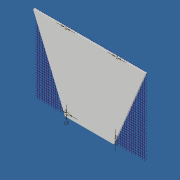
# Autodesk Inventor part: Detektorplatine
Saved by Autodesk Inventor 2018 (Build 220112000, 112)
## iProperties
Created: 2018-11-01
Part Number: Detektorplatine
Material: Generisch
Document SubType Name: Modeling
Designer: M.Knabel
Density: 1 g/cm^3
Appearance: Vorgabe
Author: M.Knabel
Autodesk Inventor part; units mm, degrees
ref_plane "YZ Plane" through (0, 0, 0) normal (1, 0, 0) x (0, 1, 0)
ref_plane "XZ Plane" through (0, 0, 0) normal (0, 1, 0) x (-1, 0, 0)
ref_plane "XY Plane" through (0, 0, 0) normal (0, 0, 1) x (1, 0, 0)
sketch "Skizze1" plane through (0, 0, 0) normal (0, 1, 0) x (-1, 0, 0)
  line L0 (-50.2277, 69) -> (50.2277, 69)
  line L1 (50.2277, 69) -> (21.647, 0)
  line L2 (21.647, 0) -> (-21.647, 0)
  line L3 (-21.647, 0) -> (-50.2277, 69)
  line L4 (0, -13.8) -> (0, 82.8) construction
  line L5 (70.3188, 0) -> (-70.3188, 0) construction
  point P0 (0, 0)
  dimension "d0" = 43.294
  dimension "d1" = 112.5
  dimension "d2" = 69
  constraints: 8 end point, 1 collinear, 1 horizontal, 1 parallel, 1 other
  measures "d0" distance of L1.end L2.end
  measures "d1" angle of L2 L3
  measures "d2" distance between parallel lines of L2 L0
extrude "Extrusion1" add sketch "Skizze1" along normal blind 1.5
sketch "Skizze2" plane through (0, 1.5, 0) normal (0, 1, 0) x (1, 0, 0)
  line L0 (21.647, 0) -> (-21.647, 0) projected
  line L1 (-21.647, 0) -> (-21.647, 7.3765) construction
  point P0 (0, 0)
  point P1 (-21.647, -1.5)
  point P2 (-19.647, -1.5)
  point P3 (-17.647, -1.5)
  point P4 (-15.647, -1.5)
  point P5 (-13.647, -1.5)
  point P6 (-11.647, -1.5)
  point P7 (-9.647, -1.5)
  point P8 (-7.647, -1.5)
  point P9 (-5.647, -1.5)
  point P10 (-3.647, -1.5)
  point P11 (-1.647, -1.5)
  point P12 (0.353, -1.5)
  point P13 (2.353, -1.5)
  point P14 (4.353, -1.5)
  point P15 (6.353, -1.5)
  point P16 (8.353, -1.5)
  point P17 (10.353, -1.5)
  point P18 (12.353, -1.5)
  point P19 (14.353, -1.5)
  point P20 (16.353, -1.5)
  point P21 (18.353, -1.5)
  point P22 (20.353, -1.5)
  point P23 (22.353, -1.5)
  point P24 (22.353, -3.5)
  point P25 (20.353, -3.5)
  point P26 (18.353, -3.5)
  point P27 (16.353, -3.5)
  point P28 (14.353, -3.5)
  point P29 (12.353, -3.5)
  point P30 (10.353, -3.5)
  point P31 (8.353, -3.5)
  point P32 (6.353, -3.5)
  point P33 (4.353, -3.5)
  point P34 (2.353, -3.5)
  point P35 (0.353, -3.5)
  point P36 (-1.647, -3.5)
  point P37 (-3.647, -3.5)
  point P38 (-5.647, -3.5)
  point P39 (-7.647, -3.5)
  point P40 (-9.647, -3.5)
  point P41 (-11.647, -3.5)
  point P42 (-13.647, -3.5)
  point P43 (-15.647, -3.5)
  point P44 (-17.647, -3.5)
  point P45 (-19.647, -3.5)
  point P46 (-21.647, -3.5)
  point P47 (22.353, -5.5)
  point P48 (20.353, -5.5)
  point P49 (18.353, -5.5)
  point P50 (16.353, -5.5)
  point P51 (14.353, -5.5)
  point P52 (12.353, -5.5)
  point P53 (10.353, -5.5)
  point P54 (8.353, -5.5)
  point P55 (6.353, -5.5)
  point P56 (4.353, -5.5)
  point P57 (2.353, -5.5)
  point P58 (0.353, -5.5)
  point P59 (-1.647, -5.5)
  point P60 (-3.647, -5.5)
  point P61 (-5.647, -5.5)
  point P62 (-7.647, -5.5)
  point P63 (-9.647, -5.5)
  point P64 (-11.647, -5.5)
  point P65 (-13.647, -5.5)
  point P66 (-15.647, -5.5)
  point P67 (-17.647, -5.5)
  point P68 (-19.647, -5.5)
  point P69 (-21.647, -5.5)
  point P70 (22.353, -7.5)
  point P71 (20.353, -7.5)
  point P72 (18.353, -7.5)
  point P73 (16.353, -7.5)
  point P74 (14.353, -7.5)
  point P75 (12.353, -7.5)
  point P76 (10.353, -7.5)
  point P77 (8.353, -7.5)
  point P78 (6.353, -7.5)
  point P79 (4.353, -7.5)
  point P80 (2.353, -7.5)
  point P81 (0.353, -7.5)
  point P82 (-1.647, -7.5)
  point P83 (-3.647, -7.5)
  point P84 (-5.647, -7.5)
  point P85 (-7.647, -7.5)
  point P86 (-9.647, -7.5)
  point P87 (-11.647, -7.5)
  point P88 (-13.647, -7.5)
  point P89 (-15.647, -7.5)
  point P90 (-17.647, -7.5)
  point P91 (-19.647, -7.5)
  point P92 (-21.647, -7.5)
  point P93 (22.353, -9.5)
  point P94 (20.353, -9.5)
  point P95 (18.353, -9.5)
  point P96 (16.353, -9.5)
  point P97 (14.353, -9.5)
  point P98 (12.353, -9.5)
  point P99 (10.353, -9.5)
  point P100 (8.353, -9.5)
  point P101 (6.353, -9.5)
  point P102 (4.353, -9.5)
  point P103 (2.353, -9.5)
  point P104 (0.353, -9.5)
  point P105 (-1.647, -9.5)
  point P106 (-3.647, -9.5)
  point P107 (-5.647, -9.5)
  point P108 (-7.647, -9.5)
  point P109 (-9.647, -9.5)
  point P110 (-11.647, -9.5)
  point P111 (-13.647, -9.5)
  point P112 (-15.647, -9.5)
  point P113 (-17.647, -9.5)
  point P114 (-19.647, -9.5)
  point P115 (-21.647, -9.5)
  point P116 (22.353, -11.5)
  point P117 (20.353, -11.5)
  point P118 (18.353, -11.5)
  point P119 (16.353, -11.5)
  point P120 (14.353, -11.5)
  point P121 (12.353, -11.5)
  point P122 (10.353, -11.5)
  point P123 (8.353, -11.5)
  point P124 (6.353, -11.5)
  point P125 (4.353, -11.5)
  point P126 (2.353, -11.5)
  point P127 (0.353, -11.5)
  point P128 (-1.647, -11.5)
  point P129 (-3.647, -11.5)
  point P130 (-5.647, -11.5)
  point P131 (-7.647, -11.5)
  point P132 (-9.647, -11.5)
  point P133 (-11.647, -11.5)
  point P134 (-13.647, -11.5)
  point P135 (-15.647, -11.5)
  point P136 (-17.647, -11.5)
  point P137 (-19.647, -11.5)
  point P138 (-21.647, -11.5)
  point P139 (22.353, -13.5)
  point P140 (20.353, -13.5)
  point P141 (18.353, -13.5)
  point P142 (16.353, -13.5)
  point P143 (14.353, -13.5)
  point P144 (12.353, -13.5)
  point P145 (10.353, -13.5)
  point P146 (8.353, -13.5)
  point P147 (6.353, -13.5)
  point P148 (4.353, -13.5)
  point P149 (2.353, -13.5)
  point P150 (0.353, -13.5)
  point P151 (-1.647, -13.5)
  point P152 (-3.647, -13.5)
  point P153 (-5.647, -13.5)
  point P154 (-7.647, -13.5)
  point P155 (-9.647, -13.5)
  point P156 (-11.647, -13.5)
  point P157 (-13.647, -13.5)
  point P158 (-15.647, -13.5)
  point P159 (-17.647, -13.5)
  point P160 (-19.647, -13.5)
  point P161 (-21.647, -13.5)
  point P162 (22.353, -15.5)
  point P163 (20.353, -15.5)
  point P164 (18.353, -15.5)
  point P165 (16.353, -15.5)
  point P166 (14.353, -15.5)
  point P167 (12.353, -15.5)
  point P168 (10.353, -15.5)
  point P169 (8.353, -15.5)
  point P170 (6.353, -15.5)
  point P171 (4.353, -15.5)
  point P172 (2.353, -15.5)
  point P173 (0.353, -15.5)
  point P174 (-1.647, -15.5)
  point P175 (-3.647, -15.5)
  point P176 (-5.647, -15.5)
  point P177 (-7.647, -15.5)
  point P178 (-9.647, -15.5)
  point P179 (-11.647, -15.5)
  point P180 (-13.647, -15.5)
  point P181 (-15.647, -15.5)
  point P182 (-17.647, -15.5)
  point P183 (-19.647, -15.5)
  point P184 (-21.647, -15.5)
  point P185 (22.353, -17.5)
  point P186 (20.353, -17.5)
  point P187 (18.353, -17.5)
  point P188 (16.353, -17.5)
  point P189 (14.353, -17.5)
  point P190 (12.353, -17.5)
  point P191 (10.353, -17.5)
  point P192 (8.353, -17.5)
  point P193 (6.353, -17.5)
  point P194 (4.353, -17.5)
  point P195 (2.353, -17.5)
  point P196 (0.353, -17.5)
  point P197 (-1.647, -17.5)
  point P198 (-3.647, -17.5)
  point P199 (-5.647, -17.5)
  dimension "d5" = 1.5
  dimension "d8" = 2
  dimension "d15" = 2
  dimension "d22" = 2
  dimension "d29" = 2
  constraints: 3 horizontal, 2 end point, 2 vertical, 1 point on line, 1665 other
  measures "d5" distance from line of L0 point (-21.647, -1.5)
  measures "d8" distance of point (-21.647, -1.5) point (-19.647, -1.5)
  measures "d15" distance of point (22.353, -1.5) point (22.353, -3.5)
  measures "d22" distance of point (22.353, -67.5) point (24.353, -67.5)
  measures "d29" distance of point (-21.647, -67.5) point (-23.647, -67.5)
